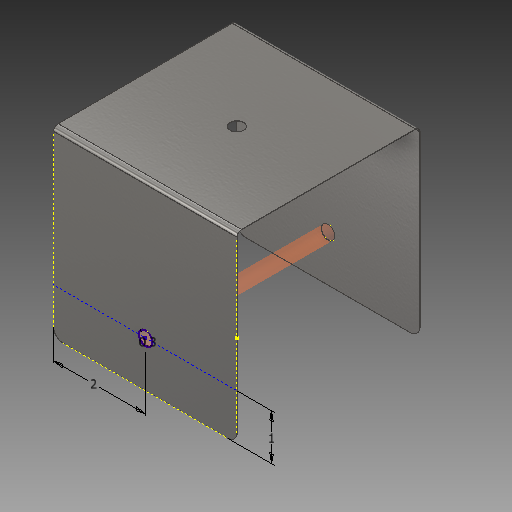
# Autodesk Inventor part: Part6
Saved by Autodesk Inventor 2019 (Build 230136000, 136)
## iProperties
Created: 2019-08-08
Part Number: Part6
Material: Steel, Galvanized
Document SubType Name: Modeling
Designer: daozhou.cen
Density: 7.85 g/cm^3
Appearance: Galvanized
Author: daozhou.cen
Autodesk Inventor part; units mm, degrees
ref_plane "YZ Plane" through (0, 0, 0) normal (1, 0, 0) x (0, 1, 0)
ref_plane "XY Plane" through (0, 0, 0) normal (0, 0, 1) x (1, 0, 0)
sketch "Sketch1" plane through (0, 0, 0) normal (1, 0, 0) x (0, 1, 0)
  line L0 (20, 20) -> (-20, 20) construction
  line L1 (-20, 20) -> (-20, -20) construction
  line L2 (-20, -20) -> (20, -20) construction
  line L3 (20, -20) -> (20, 20) construction
  line L4 (20, 20) -> (-20, -20) construction
  line L5 (-20, 20) -> (20, -20) construction
  line L6 (-20, 20) -> (19, 20)
  arc A0 (20, 19) -> (19, 20) centre (19, 19) ccw
  line L7 (-20, -20) -> (19, -20)
  arc A1 (19, -20) -> (20, -19) centre (19, -19) ccw
  line L8 (20, -19) -> (20, 19)
  point P0 (0, 0)
  dimension "d0" = 40
  dimension "d1" = 40
  dimension "d2" = 39
  dimension "d3" = 39
  constraints: 18 end point, 4 point on circle, 4 point on line, 4 tangent, 2 centre point, 2 midpoint, 2 parallel, 1 collinear, 1 horizontal, 1 perpendicular
  measures "d0" distance of L2.end L1.end
  measures "d1" distance of L1.end L0.end
  measures "d2" distance of L0.end L6.end
  measures "d3" distance of L1.end L7.end
ref_plane "Work Plane1" through (0, -20, 20) normal (0, 1, 0) x (-1, 0, 0)
sketch "Sketch2" plane through (0, -20, 20) normal (0, 1, 0) x (-1, 0, 0)
  line L0 (0, 0) -> (40, 0)
  line L1 (40, 0) -> (40, -0.1)
  line L2 (40, -0.1) -> (0, -0.1)
  line L3 (0, -0.1) -> (0, 0)
  point P0 (0, -20)
  dimension "d4" = 40
  dimension "d5" = 0.1
  constraints: 8 end point, 2 parallel, 1 horizontal, 1 perpendicular
  measures "d4" distance of L1.end L2.end
  measures "d5" distance of L0.end L1.end
sweep "Sweep1" add profiles "Sketch2" path "Sketch1" path curves L6 A0 L8 A1 L7
fillet "Fillet1" radius 2 4 edges at (0, -20, 19.95) (-40, -20, 19.95) (0, -20, -19.95) (-40, -20, -19.95)
sketch "Sketch3" plane through (-40, 19, 20) normal (0, 0, 1) x (1, 0, 0)
  circle A0 centre (20, -29) radius 1.5
  line L0 (0, 0) -> (0, -37) construction
  line L1 (0, -29) -> (40, -29) construction
  line L2 (40, 0) -> (40, -37) construction
  line L3 (38, -39) -> (2, -39) construction
  point P0 (40, -19)
  dimension "d9" = 3
  dimension "d10" = 10
  dimension "d11" = 20
  constraints: 2 end point, 2 point on line, 1 centre point, 1 horizontal, 1 midpoint
  measures "d9" diameter of A0
  measures "d10" distance between parallel lines of L1 L3
  measures "d11" distance from line of L0 A0.centre
extrude "Extrusion1" cut sketch "Sketch3" against normal through all
surface extrude "ExtrusionSrf1" sketch "Sketch3" against normal through all shown yes curves A0
sketch "Sketch4" plane through (-40, 20, 19) normal (0, 1, 0) x (1, 0, 0)
  line L0 (0, 0) -> (40, 0) construction
  line L1 (0, 38) -> (40, 38) construction
  line L2 (0, 0) -> (40, 38) construction
  line L3 (40, 0) -> (40, 38) construction
  line L4 (40, 0) -> (0, 38) construction
  point P0 (40, 19)
  point P1 (20, 19)
  constraints: 4 end point, 1 midpoint
hole "Hole1" at (-20, 20, 0) direction (0, -1, 0) diameter 3 end through all
equation "\"d3\" = d2"
body "Solid1"
body "Srf1"
